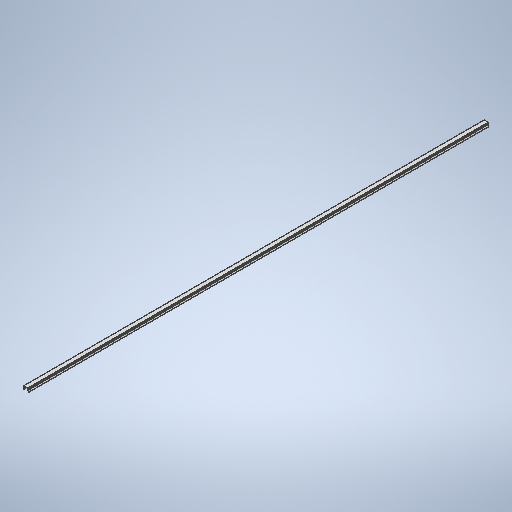
# Autodesk Inventor part: HD - 402 PERFIL ALUMINO - PASAMANOS RECTANGULAR
Saved by Autodesk Inventor 2025 (Build 290162000, 162)
## iProperties
Created: 2026-01-25
Part Number: HD - 402 PERFIL ALUMINO - PASAMANOS RECTANGULAR
Material: Generic
Document SubType Name: Modeling
Designer: Frank
Density: 1 g/cm^3
Appearance: Default
Author: Frank
Autodesk Inventor part; units mm, degrees
ref_plane "YZ Plane" through (0, 0, 0) normal (1, 0, 0) x (0, 1, 0)
ref_plane "XZ Plane" through (0, 0, 0) normal (0, 1, 0) x (-1, 0, 0)
ref_plane "XY Plane" through (0, 0, 0) normal (0, 0, 1) x (1, 0, 0)
sketch "Sketch1" plane through (0, 0, 0) normal (0, 0, 1) x (1, 0, 0)
  line L0 (-19.8968, 26.095) -> (1.1032, 26.095)
  line L1 (10.1032, 18.595) -> (10.1032, -13.405)
  line L2 (9.6032, -13.905) -> (6.1032, -13.905)
  line L3 (-19.8968, 24.095) -> (0.6032, 24.095)
  line L4 (7.6032, -11.905) -> (6.1032, -11.905)
  line L5 (3.1032, 24.095) -> (3.1032, 19.595)
  line L6 (3.6032, 19.095) -> (9.6032, 19.095)
  line L7 (-19.8968, 31.6782) -> (-19.8968, -20.1233) construction
  line L8 (1.1032, 23.595) -> (1.1032, 17.595)
  line L9 (1.1032, 17.095) -> (1.1032, 17.095)
  line L10 (7.6032, 17.095) -> (1.6032, 17.095)
  line L11 (7.6032, 9.395) -> (0.6032, 9.395)
  line L12 (0.1032, 8.895) -> (0.1032, -1.105)
  line L13 (0.6032, -1.605) -> (1.4032, -1.605)
  line L14 (2.4032, 7.595) -> (7.6032, 7.595)
  line L15 (2.7032, 3.7552) -> (1.9032, 4.2999)
  line L16 (2.7032, 3.7552) -> (1.9032, 3.306)
  line L17 (1.9032, -1.105) -> (1.9032, 3.306)
  line L18 (1.9032, 4.2999) -> (1.9032, 7.095)
  line L19 (5.6032, -13.405) -> (5.6032, -12.405)
  line L20 (8.1032, 16.595) -> (8.1032, 9.895)
  line L21 (8.1032, 7.095) -> (8.1032, -11.405)
  arc A0 (3.1032, 24.095) -> (1.1032, 26.095) centre (1.1032, 24.095) ccw
  arc A1 (1.1032, 17.595) -> (1.6032, 17.095) centre (1.6032, 17.595) ccw
  arc A2 (3.1032, 19.595) -> (3.6032, 19.095) centre (3.6032, 19.595) ccw
  arc A3 (10.1032, 18.595) -> (9.6032, 19.095) centre (9.6032, 18.595) ccw
  arc A4 (7.6032, 9.395) -> (8.1032, 9.895) centre (7.6032, 9.895) ccw
  arc A5 (8.1032, 7.095) -> (7.6032, 7.595) centre (7.6032, 7.095) ccw
  arc A6 (0.6032, 9.395) -> (0.1032, 8.895) centre (0.6032, 8.895) ccw
  arc A7 (0.1032, -1.105) -> (0.6032, -1.605) centre (0.6032, -1.105) ccw
  arc A8 (1.4032, -1.605) -> (1.9032, -1.105) centre (1.4032, -1.105) ccw
  arc A9 (2.4032, 7.595) -> (1.9032, 7.095) centre (2.4032, 7.095) ccw
  arc A10 (8.1032, 16.595) -> (7.6032, 17.095) centre (7.6032, 16.595) ccw
  arc A11 (7.6032, -11.905) -> (8.1032, -11.405) centre (7.6032, -11.405) ccw
  arc A12 (6.1032, -11.905) -> (5.6032, -12.405) centre (6.1032, -12.405) ccw
  arc A13 (5.6032, -13.405) -> (6.1032, -13.905) centre (6.1032, -13.405) ccw
  arc A14 (9.6032, -13.905) -> (10.1032, -13.405) centre (9.6032, -13.405) ccw
  arc A15 (1.1032, 23.595) -> (0.6032, 24.095) centre (0.6032, 23.595) ccw
  line L22 (-19.8968, 26.095) -> (-40.8968, 26.095)
  line L23 (-49.8968, 18.595) -> (-49.8968, -13.405)
  line L24 (-49.3968, -13.905) -> (-45.8968, -13.905)
  line L25 (-19.8968, 24.095) -> (-40.3968, 24.095)
  line L26 (-47.3968, -11.905) -> (-45.8968, -11.905)
  line L27 (-42.8968, 24.095) -> (-42.8968, 19.595)
  line L28 (-43.3968, 19.095) -> (-49.3968, 19.095)
  line L29 (-40.8968, 23.595) -> (-40.8968, 17.595)
  line L30 (-40.8968, 17.095) -> (-40.8968, 17.095)
  line L31 (-47.3968, 17.095) -> (-41.3968, 17.095)
  line L32 (-47.3968, 9.395) -> (-40.3968, 9.395)
  line L33 (-39.8968, 8.895) -> (-39.8968, -1.105)
  line L34 (-40.3968, -1.605) -> (-41.1968, -1.605)
  line L35 (-42.1968, 7.595) -> (-47.3968, 7.595)
  line L36 (-42.4968, 3.7552) -> (-41.6968, 4.2999)
  line L37 (-42.4968, 3.7552) -> (-41.6968, 3.306)
  line L38 (-41.6968, -1.105) -> (-41.6968, 3.306)
  line L39 (-41.6968, 4.2999) -> (-41.6968, 7.095)
  line L40 (-45.3968, -13.405) -> (-45.3968, -12.405)
  line L41 (-47.8968, 16.595) -> (-47.8968, 9.895)
  line L42 (-47.8968, 7.095) -> (-47.8968, -11.405)
  arc A16 (-40.8968, 26.095) -> (-42.8968, 24.095) centre (-40.8968, 24.095) ccw
  arc A17 (-41.3968, 17.095) -> (-40.8968, 17.595) centre (-41.3968, 17.595) ccw
  arc A18 (-43.3968, 19.095) -> (-42.8968, 19.595) centre (-43.3968, 19.595) ccw
  arc A19 (-49.3968, 19.095) -> (-49.8968, 18.595) centre (-49.3968, 18.595) ccw
  arc A20 (-47.8968, 9.895) -> (-47.3968, 9.395) centre (-47.3968, 9.895) ccw
  arc A21 (-47.3968, 7.595) -> (-47.8968, 7.095) centre (-47.3968, 7.095) ccw
  arc A22 (-39.8968, 8.895) -> (-40.3968, 9.395) centre (-40.3968, 8.895) ccw
  arc A23 (-40.3968, -1.605) -> (-39.8968, -1.105) centre (-40.3968, -1.105) ccw
  arc A24 (-41.6968, -1.105) -> (-41.1968, -1.605) centre (-41.1968, -1.105) ccw
  arc A25 (-41.6968, 7.095) -> (-42.1968, 7.595) centre (-42.1968, 7.095) ccw
  arc A26 (-47.3968, 17.095) -> (-47.8968, 16.595) centre (-47.3968, 16.595) ccw
  arc A27 (-47.8968, -11.405) -> (-47.3968, -11.905) centre (-47.3968, -11.405) ccw
  arc A28 (-45.3968, -12.405) -> (-45.8968, -11.905) centre (-45.8968, -12.405) ccw
  arc A29 (-45.8968, -13.905) -> (-45.3968, -13.405) centre (-45.8968, -13.405) ccw
  arc A30 (-49.8968, -13.405) -> (-49.3968, -13.905) centre (-49.3968, -13.405) ccw
  arc A31 (-40.3968, 24.095) -> (-40.8968, 23.595) centre (-40.3968, 23.595) ccw
  point P0 (0, 0)
  point P1 (6.6032, 19.095)
  point P2 (4.1032, 9.395)
  point P3 (1.0032, -1.605)
  point P4 (5.6032, -12.905)
  point P5 (7.8532, -13.905)
  point P6 (1.9032, 5.6974)
  point P7 (-39.7937, 0)
  point P8 (-46.3968, 19.095)
  point P9 (-43.8968, 9.395)
  point P10 (-40.7968, -1.605)
  point P11 (-45.3968, -12.905)
  point P12 (-47.6468, -13.905)
  point P13 (-41.6968, 5.6974)
  dimension "d4" = 7
  dimension "d5" = 7
  dimension "d6" = 2
  dimension "d7" = 2
  dimension "d9" = 2
  dimension "d11" = 7.7
  dimension "d12" = 1.8
  dimension "d14" = 11
  dimension "d16" = 4.5
  dimension "d17" = 2
  dimension "d20" = 0.5
  dimension "d22" = 40
  dimension "d23" = 1.8
  dimension "d24" = 60
  constraints: 86 end point, 64 point on circle, 59 symmetric about line, 32 centre point, 32 tangent, 13 equal radius, 11 perpendicular, 6 midpoint, 6 point on line, 4 parallel, 3 horizontal, 16 other
  measures "d4" distance between parallel lines of L1 L5
  measures "d5" distance from line of L0 point (6.603, 19.095)
  measures "d6" distance between parallel lines of L5 L8
  measures "d7" distance between parallel lines of L10 L6
  measures "d9" distance between parallel lines of L4 L2
  measures "d11" distance between parallel lines of L11 L10
  measures "d12" distance from line of point (4.103, 9.395) L14
  measures "d14" distance from line of L11 point (1.003, -1.605)
  measures "d16" distance from line of L1 point (5.603, -12.905)
  measures "d17" radius of A0
  measures "d20" radius of A15
  measures "d22" distance from line of point (7.853, -13.905) L0
  measures "d23" distance from line of L12 point (1.903, 5.697)
  measures "d24" distance between parallel lines of L1 L23
extrude "Extrusion1" add sketch "Sketch1" against normal blind 5000
body "Solid1"
